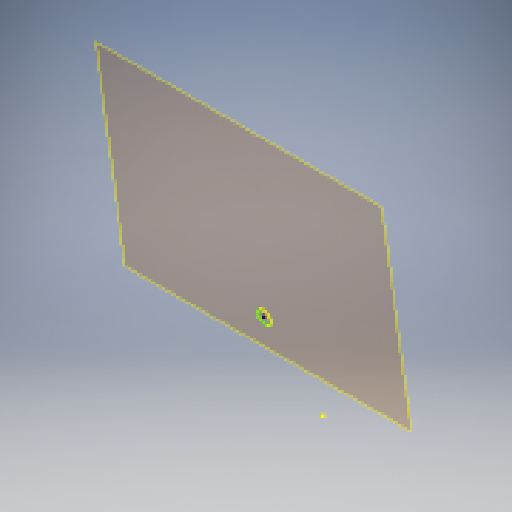
# Autodesk Inventor part: Part1
Saved by Autodesk Inventor 2024 (Build 280153000, 153)
## iProperties
Created: 2025-01-10
Part Number: Part1
Material: Generic
Document SubType Name: Modeling
Designer: Alex
Density: 1 g/cm^3
Appearance: Default
Author: Alex
Autodesk Inventor part; units mm, degrees
ref_plane "YZ Plane" through (0, 0, 0) normal (1, 0, 0) x (0, 1, 0)
ref_plane "XZ Plane" through (0, 0, 0) normal (0, 1, 0) x (-1, 0, 0)
ref_plane "XY Plane" through (0, 0, 0) normal (0, 0, 1) x (1, 0, 0)
ref_plane "Work Plane1" through (46.4934, 164.1502, -100.8153) normal (0, -0.1396054, 0.9902072) x (1, 0, 0)
sketch "Sketch1" plane through (46.4934, 164.1502, -100.8153) normal (0, -0.1396054, 0.9902072) x (1, 0, 0)
  circle A0 centre (-77.9553, -107.0952) radius 4.3235 projected
  circle A1 centre (-77.9553, -107.0952) radius 4.1018
  point P0 (-46.4934, -148.4684)
  constraints: 1 centre point, 1 coincident
extrude "Extrusion1" add sketch "Sketch1" against normal blind 25.4 contours A1
thread "Thread1" size "3/8-16 UNC" class "2A" standard "ANSI Unified Screw Threads" length 11
sketch "Sketch2" plane through (46.4934, 164.1502, -100.8153) normal (0, -0.1396054, 0.9902072) x (1, 0, 0)
  circle A0 centre (-77.9553, -107.0952) radius 4.3235 construction
  line L0 (0, -50.1427) -> (0, 0) construction
  arc A1 (-38.2285, -91.2202) -> (0, -50.1427) centre (-77.9553, -15.9215) ccw construction
  line L1 (-38.2285, -91.2202) -> (-117.6821, -91.2202) construction
  arc A2 (-155.9106, -50.1427) -> (-117.6821, -91.2202) centre (-77.9553, -15.9215) ccw construction
  line L2 (-155.9106, -50.1427) -> (-155.9106, 0) construction
  line L3 (-155.9106, 0) -> (-159.0856, 0) construction
  line L4 (-159.0856, -50.1427) -> (-159.0856, 0) construction
  arc A3 (-159.0856, -50.1427) -> (-117.8938, -94.3952) centre (-77.9553, -15.9215) ccw construction
  line L5 (-117.8938, -94.3952) -> (-103.6066, -94.3952) construction
  line L6 (-103.6066, -94.3952) -> (-103.6066, -119.7952) construction
  line L7 (-52.304, -119.7952) -> (-103.6066, -119.7952) construction
  line L8 (-52.304, -94.3952) -> (-52.304, -119.7952) construction
  line L9 (-52.304, -94.3952) -> (-38.0167, -94.3952) construction
  arc A4 (-38.0167, -94.3952) -> (3.175, -50.1427) centre (-77.9553, -15.9215) ccw construction
  line L10 (3.175, 0) -> (3.175, -50.1427) construction
  line L11 (0, 0) -> (3.175, 0) construction
  line L12 (-96.3354, -100.2936) -> (-59.5752, -100.2936)
  line L13 (-59.5752, -100.2936) -> (-59.5752, -113.8968)
  line L14 (-59.5752, -113.8968) -> (-96.3354, -113.8968)
  line L15 (-96.3354, -113.8968) -> (-96.3354, -100.2936)
  line L16 (-96.3354, -107.0952) -> (-59.5752, -107.0952) construction
  line L17 (-77.9553, -100.2936) -> (-77.9553, -113.8968) construction
  point P0 (-46.4934, -148.4684)
  constraints: 12 end point, 5 midpoint, 2 coincident, 2 parallel, 1 horizontal, 1 perpendicular
extrude "Extrusion2" add sketch "Sketch2" along normal blind 6.35
sketch "Sketch4" plane through (-49.842, 51.3688, -116.7159) normal (0, -0.9902072, -0.1396054) x (1, 0, 0)
  line L0 (0, 0) -> (36.7602, 0) construction
  line L1 (36.7602, 0) -> (36.7602, 6.35) construction
  line L2 (0, 6.35) -> (36.7602, 6.35) construction
  line L3 (0, 0) -> (0, 6.35) construction
  line L4 (0, 15.2304) -> (36.7602, 15.2304) construction
  line L5 (36.7602, 21.5804) -> (0, 21.5804) construction
  line L6 (0, 21.5804) -> (0, 15.2304) construction
  line L7 (30.4102, 59.9083) -> (30.4102, 21.5804) construction
  line L8 (0, 30.4608) -> (30.4102, 30.4608) construction
  line L9 (0, 30.4608) -> (0, 36.8108) construction
  line L10 (6.35, 6.35) -> (6.35, 15.2304) construction
  line L11 (36.7602, 36.8108) -> (0, 36.8108) construction
  line L12 (0, 30.4608) -> (0, 36.8108) construction
  line L13 (36.7602, 15.2304) -> (36.7602, 36.8108) construction
  line L14 (0, 0) -> (0, 21.5804) construction
  line L15 (6.35, 6.35) -> (6.35, 15.2304)
  line L16 (6.35, 15.2304) -> (36.7602, 15.2304)
  line L17 (36.7602, 15.2304) -> (36.7602, 36.8108)
  line L18 (0, 36.8108) -> (36.7602, 36.8108)
  line L19 (0, 36.8108) -> (0, 30.4608)
  line L20 (0, 30.4608) -> (30.4102, 30.4608)
  line L21 (30.4102, 30.4608) -> (30.4102, 21.5804)
  line L22 (30.4102, 21.5804) -> (0, 21.5804)
  line L23 (0, 21.5804) -> (0, 6.35)
  line L24 (0, 6.35) -> (6.35, 6.35)
  line L25 (0, 6.35) -> (36.7602, 6.35) projected
  point P0 (49.842, 122.7443)
  dimension "d7" = 6.35
  dimension "d11" = 6.35
  dimension "d12" = 6.35
  dimension "d13" = 6.35
  constraints: 42 end point, 10 collinear, 6 point on line, 5 perpendicular, 3 vertical, 2 parallel, 1 horizontal
  measures "d7" distance between parallel lines of L5 L4
  measures "d11" distance between parallel lines of L10 L14
  measures "d12" distance between parallel lines of L13 L7
  measures "d13" distance between parallel lines of L11 L8
extrude "Extrusion3" add sketch "Sketch4" against normal up to surface (13.6032 mm away)
sketch "Sketch5" plane through (-49.842, 46.2298, -80.2656) normal (0, -0.1396054, 0.9902072) x (1, 0, 0)
  circle A0 centre (18.3801, 6.8016) radius 4.1018 projected
  point P0 (49.842, -34.5716)
extrude "Extrusion4" cut sketch "Sketch5" against normal up to surface (6.35 mm away)
body "Solid1"
